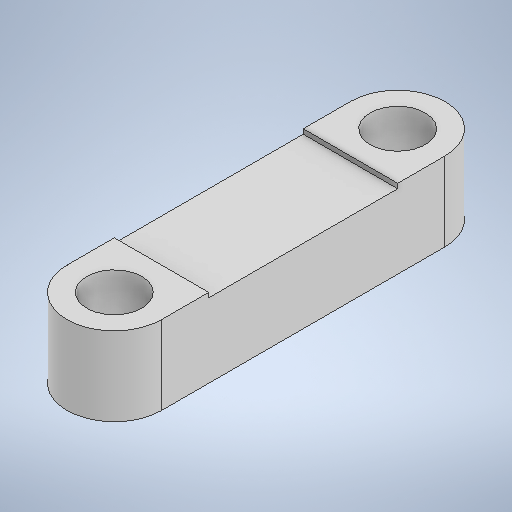
# Autodesk Inventor part: Belt Holder
Saved by Autodesk Inventor 2026.2 (Build 302298010, 298A)
## iProperties
Created: 2026-05-02
Part Number: Belt Holder
Material: Generic
Document SubType Name: Modeling
Designer: piete
Density: 1 g/cm^3
Appearance: Default
Author: piete
Autodesk Inventor part; units mm, degrees
ref_plane "YZ Plane" through (0, 0, 0) normal (1, 0, 0) x (0, 1, 0)
ref_plane "XZ Plane" through (0, 0, 0) normal (0, 1, 0) x (-1, 0, 0)
ref_plane "XY Plane" through (0, 0, 0) normal (0, 0, 1) x (1, 0, 0)
sketch "Sketch1" plane through (0, 0, 0) normal (0, 1, 0) x (-1, 0, 0)
  circle A0 centre (0, 9) radius 1.75
  circle A1 centre (0, -9) radius 1.75
  circle A2 centre (0, 9) radius 3
  circle A3 centre (0, -9) radius 3
  line L0 (3, 9) -> (-3, 9)
  line L1 (-3, 9) -> (-3, -9)
  line L2 (-3, -9) -> (3, -9)
  line L3 (3, -9) -> (3, 9)
  point P0 (0, 0)
  point P1 (-3, 9)
  point P2 (3, -9)
  dimension "d6" = 6
  dimension "d7" = 6
  dimension "d0" = 3.5
  dimension "d1" = 3.5
  dimension "d2" = 9
  dimension "d3" = 9
  dimension "d4" = 0
  dimension "d5" = 0
  dimension "d8" = 18
  dimension "d9" = 6
  constraints: 8 end point, 2 centre point, 2 coincident, 2 parallel, 1 horizontal, 1 perpendicular, 6 other
  measures "d0" diameter of A0
  measures "d1" diameter of A1
  measures "d2" distance of point (0, 0) A1.centre
  measures "d3" distance of point (0, 0) A0.centre
  measures "d4" horizontal distance of point (0, 0) A0.centre
  measures "d5" horizontal distance of point (0, 0) A1.centre
  measures "d8" distance of L2.end L0.start
  measures "d9" distance of L0.start L0.end
extrude "Extrusion1" add sketch "Sketch1" along normal blind 5 contours L0 A2 A0 | A0 L0 A2 | L3 A3 L1 A2 | L2 A1 A3 | A3 L2 A1
sketch "Sketch2" plane through (0, 5, 0) normal (0, 1, 0) x (1, 0, 0)
  line L0 (-3, 9) -> (-3, -9) projected
  line L1 (3, -9) -> (3, 9) projected
  line L2 (-3, -6) -> (3, -6)
  line L3 (3, -6) -> (3, 6)
  line L4 (3, 6) -> (-3, 6)
  line L5 (-3, 6) -> (-3, -6)
  point P0 (0, 0)
  point P1 (3, -6)
  dimension "d12" = 6
  dimension "d13" = 6
  constraints: 8 end point, 2 parallel, 2 point on line, 1 horizontal, 1 perpendicular
  measures "d12" distance from line of point (0, 0) L4
  measures "d13" distance from line of point (0, 0) L2
extrude "Extrusion2" cut sketch "Sketch2" against normal blind 0.3
body "Solid1"
